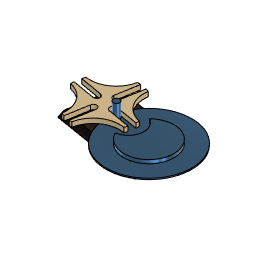
cool_old_stuffff (Autodesk Fusion 360 design; units mm, degrees)
Autodesk Fusion 360 part; units mm, degrees
sketch "Sketch1" plane through (0, 0, 0) normal (0, 0, 1) x (1, 0, 0)
  line L0 (70, 40) -> (-70, 40)
  line L1 (-70, 40) -> (-70, -40)
  line L2 (-70, -40) -> (70, -40)
  line L3 (70, -40) -> (70, 40)
  line L4 (70, 40) -> (-70, -40) construction
  line L5 (-70, 40) -> (70, -40) construction
  constraint horizontal L0
  constraint perpendicular L0 L1
  constraint parallel L0 L2
  constraint parallel L1 L3
  constraint coincident L4 origin
  constraint coincident L5 origin
ref_plane "WorkPlane1" through (0, 0, 10) normal (0, 0, 1) x (1, 0, 0)
sketch "Sketch2" plane through (0, 0, 10) normal (0, 0, 1) x (1, 0, 0)
  line L0 (65, -35) -> (-65, -35)
  line L1 (-65, -35) -> (-65, 35)
  line L2 (-65, 35) -> (65, 35)
  line L3 (65, 35) -> (65, -35)
  line L4 (65, -35) -> (-65, 35) construction
  line L5 (-65, -35) -> (65, 35) construction
  constraint horizontal L0
  constraint perpendicular L0 L1
  constraint parallel L0 L2
  constraint parallel L1 L3
  constraint coincident L4 origin
  constraint coincident L5 origin
loft "Loft1" add profiles "Sketch1", "Sketch2" section 1 section 2 makes body 1
sketch "Sketch3" plane through (0, 0, 10) normal (0, 0, 1) x (-1, 0, 0)
  line L0 (-65, 35) -> (-65, -35)
  line L1 (-65, -35) -> (65, -35)
  line L2 (65, -35) -> (65, 35)
  line L3 (65, 35) -> (-65, 35)
  circle A0 centre (40, 0) radius 7.5
  circle A1 centre (-40, 0) radius 7.5
  dimension "d2" = 15
  dimension "d3" = 15
  measures "d2" diameter of A0
  measures "d3" diameter of A1
extrude "Extrude1" cut sketch "Sketch3" against normal blind 35 contours A0 | A1 bodies 1
sketch "Sketch5" plane through (0, 0, 10) normal (0, 0, 1) x (1, 0, 0)
  line L0 (-54.9257, 4.9994) -> (-89.7494, 4.9994)
  line L1 (-54.9257, -4.9994) -> (-89.7494, -4.9994)
  line L2 (-44.9992, 14.9113) -> (-44.9992, 49.7495)
  line L3 (-35.0008, 14.9113) -> (-35.0008, 49.7495)
  line L4 (-25.0347, 4.9999) -> (9.7494, 4.9999)
  line L5 (-25.0347, -4.9999) -> (9.7494, -4.9999)
  line L6 (-35.0004, -14.9355) -> (-35.0004, -49.7494)
  line L7 (-44.9996, -14.9355) -> (-44.9996, -49.7494)
  arc A0 (-55.0743, -4.9994) -> (-55.0743, 4.9994) centre (-55, 0) ccw
  arc A1 (-44.9992, 15.0887) -> (-35.0008, 15.0887) centre (-40, 15) ccw
  arc A2 (-24.9653, 4.9999) -> (-24.9653, -4.9999) centre (-25, 0) ccw
  arc A3 (-35.0004, -15.0645) -> (-44.9996, -15.0645) centre (-40, -15) ccw
  line L8 (-44.9996, -49.7494) -> (-104, -49) construction
  line L9 (-104, -49) -> (-93.0357, -49.1393) construction
  line L10 (-89.7494, -4.9994) -> (-89.7494, -49.181) construction
  line L11 (-89.7494, 4.9994) -> (-89.7494, 62) construction
  line L12 (-89.7494, 62) -> (-72.3376, 62) construction
  line L13 (-72.3376, 62) -> (-89.7494, 58.8778) construction
  line L14 (-53.6946, 49.7495) -> (-91, 49.7495) construction
  line L15 (-91, 49.7495) -> (-87, 49.7495) construction
  line L16 (-35.0008, 49.7495) -> (24, 49.7495) construction
  line L17 (24, 49.7495) -> (20, 49.7495) construction
  line L18 (9.7494, 4.9999) -> (10, 52) construction
  line L19 (10, 52) -> (9.988, 49.7495) construction
  line L20 (9.7494, -4.9999) -> (9.7494, -65) construction
  line L21 (9.7494, -65) -> (9.7494, -62) construction
  line L22 (-35.0004, -49.7494) -> (11, -49.7494) construction
  line L23 (11, -49.7494) -> (9.7494, -49.7494) construction
  arc A4 (-49.7527, -49.689) -> (-89.7494, -9.181) centre (-89.7494, -49.181) ccw
  arc A5 (-89.7494, -4.9994) -> (-89.149, -9.1855) centre (-40, 0) ccw
  arc A6 (-49.7497, -49.0402) -> (-44.9996, -49.7494) centre (-40, 0) ccw
  arc A7 (-89.7494, 9.7495) -> (-49.7557, 49.039) centre (-89.7494, 49.7495) ccw
  arc A8 (-44.9992, 49.7495) -> (-49.7557, 49.039) centre (-40, 0) ccw
  arc A9 (-89.039, 9.7558) -> (-89.7494, 4.9994) centre (-40, 0) ccw
  arc A10 (-30.012, 49.7495) -> (9.7747, 9.75) centre (9.988, 49.7495) ccw
  arc A11 (9.7494, 4.9999) -> (9.038, 9.7607) centre (-40, 0) ccw
  arc A12 (-30.0048, 48.9908) -> (-35.0008, 49.7495) centre (-40, 0) ccw
  arc A13 (9.7494, -9.7494) -> (-30.2506, -49.7494) centre (9.7494, -49.7494) ccw
  arc A14 (-35.0004, -49.7494) -> (-30.2443, -49.039) centre (-40, 0) ccw
  arc A15 (9.039, -9.7557) -> (9.7494, -4.9999) centre (-40, 0) ccw
  dimension "d15" = 100
  dimension "d16" = 10
  dimension "d17" = 10
  dimension "d18" = 10
  dimension "d19" = 10
  dimension "d20" = 80
  dimension "d21" = 80
  dimension "d22" = 80
  dimension "d23" = 80
  constraint coincident L0.start A0
  constraint horizontal L0
  constraint coincident L1.start A0
  constraint parallel L0 L1
  constraint coincident L2.start A1
  constraint coincident L2.end A5
  constraint perpendicular L1 L2
  constraint coincident L3.start A1
  constraint parallel L2 L3
  constraint coincident L4.start A2
  constraint coincident L4.end A5
  constraint perpendicular L3 L4
  constraint coincident L5.start A2
  constraint perpendicular L3 L5
  constraint coincident L6.start A3
  constraint coincident L6.end A5
  constraint perpendicular L0 L6
  constraint coincident L7.start A3
  constraint parallel L6 L7
  constraint coincident L0 A0.end
  constraint coincident L1 A0.start
  constraint coincident L3 A1.end
  constraint coincident L2 A1.start
  constraint concentric A5 A8
  constraint coincident L5 A2.end
  constraint coincident L4 A2.start
  constraint concentric A5 A11
  constraint coincident L7 A3.end
  constraint coincident L6 A3.start
  constraint concentric A5 A14
  constraint coincident L8 L9.end
  constraint parallel L8 L9
  constraint coincident L8 L10.end
  constraint perpendicular L1 L10
  constraint perpendicular L0 L11
  constraint perpendicular L11 L12
  constraint coincident L11 L13.end
  constraint perpendicular L11 L14
  constraint coincident L14 L15.end
  constraint perpendicular L11 L15
  constraint perpendicular L3 L16
  constraint coincident L16 L17.end
  constraint perpendicular L3 L17
  constraint coincident L18 L19.end
  constraint coincident L16 L19.end
  constraint parallel L18 L19
  constraint perpendicular L5 L20
  constraint coincident L20 L21.end
  constraint perpendicular L5 L21
  constraint perpendicular L20 L22
  constraint coincident L22 L23.end
  constraint coincident L20 L23.end
  constraint perpendicular L20 L23
  constraint coincident L10.end A4.centre
  constraint coincident L14 A7.centre
  constraint coincident L11 A7.centre
  constraint coincident L19.end A10.centre
  constraint coincident L10 A4.end
  constraint coincident L8 A4.start
  constraint coincident A4 A5.end
  constraint coincident A4 A6.start
  constraint concentric A5 A6
  constraint coincident L11 A7.start
  constraint coincident A7 A9.start
  constraint concentric A8 A9
  constraint coincident L18 A10.end
  constraint coincident L16 A10.start
  constraint coincident A10 A11.end
  constraint coincident A10 A12.start
  constraint concentric A11 A12
  constraint coincident L23.end A13.centre
  constraint coincident L22 A13.end
  constraint coincident L20 A13.start
  constraint coincident A13 A14.end
  constraint coincident A13 A15.start
  constraint concentric A14 A15
  measures "d15" diameter of A5
  measures "d16" diameter of A0
  measures "d17" diameter of A1
  measures "d18" diameter of A2
  measures "d19" diameter of A3
  measures "d20" diameter of A4
  measures "d21" diameter of A7
  measures "d22" diameter of A10
  measures "d23" diameter of A13
ref_plane "WorkPlane3" through (0, 0, 20) normal (0, 0, 1) x (-1, 0, 0)
sketch "Sketch7" plane through (0, 0, 20) normal (0, 0, 1) x (1, 0, 0)
  line L0 (-54.7838, 4.9953) -> (-89.7498, 4.9953)
  line L1 (-54.7838, -4.9953) -> (-89.7498, -4.9953)
  line L2 (-44.998, 15.1402) -> (-44.998, 49.7496)
  line L3 (-35.002, 15.1402) -> (-35.002, 49.7496)
  line L4 (-24.9087, 4.9992) -> (9.7495, 4.9992)
  line L5 (-24.9087, -4.9992) -> (9.7495, -4.9992)
  line L6 (-45, -14.9847) -> (-45.1061, -49.7386)
  line L7 (-35, -14.9847) -> (-34.8939, -49.7386)
  arc A0 (-88.9872, 10.0128) -> (-50.0128, 48.9872) centre (-90, 50) ccw
  arc A1 (-44.998, 49.7496) -> (-50.0128, 48.9872) centre (-40, 0) ccw
  arc A2 (-44.998, 15.1402) -> (-35.002, 15.1402) centre (-40, 15) ccw
  arc A3 (-29.9872, 48.9872) -> (8.9872, 10.0128) centre (10, 50) ccw
  arc A4 (-29.9872, 48.9872) -> (-35.002, 49.7496) centre (-40, 0) ccw
  arc A5 (9.7495, 4.9992) -> (8.9872, 10.0128) centre (-40, 0) ccw
  arc A6 (-24.9087, 4.9992) -> (-24.9087, -4.9992) centre (-25, 0) ccw
  arc A7 (8.9872, -10.0128) -> (-29.9872, -48.9872) centre (10, -50) ccw
  arc A8 (8.9872, -10.0128) -> (9.7495, -4.9992) centre (-40, 0) ccw
  arc A9 (-34.8939, -49.7386) -> (-29.9872, -48.9872) centre (-40, 0) ccw
  arc A10 (-35, -14.9847) -> (-45, -14.9847) centre (-40, -15) ccw
  arc A11 (-50, -48.9898) -> (-89.1818, -9.0084) centre (-90, -49) ccw
  arc A12 (-50, -48.9898) -> (-45.1061, -49.7386) centre (-40, 0) ccw
  arc A13 (-88.9872, 10.0128) -> (-89.7498, 4.9953) centre (-40, 0) ccw
  arc A14 (-89.7498, -4.9953) -> (-89.1818, -9.0084) centre (-40, 0) ccw
  arc A15 (-55.2162, -4.9953) -> (-55.2162, 4.9953) centre (-55, 0) ccw
  dimension "d25" = 100
  dimension "d26" = 80
  dimension "d27" = 80
  dimension "d28" = 80
  dimension "d29" = 80
  dimension "d30" = 10
  dimension "d31" = 10
  dimension "d32" = 10
  dimension "d33" = 10
  constraint coincident L0.start A15
  constraint horizontal L0
  constraint coincident L1.start A15
  constraint coincident L1.end A13
  constraint parallel L0 L1
  constraint coincident L2.end A13
  constraint perpendicular L0 L2
  constraint parallel L2 L3
  constraint coincident L4.end A13
  constraint perpendicular L3 L4
  constraint parallel L4 L5
  constraint tangent L6 A10
  constraint coincident L7.end A13
  constraint tangent L7 A10
  constraint concentric A1 A13
  constraint coincident A3.start A13
  constraint concentric A4 A13
  constraint concentric A5 A13
  constraint coincident A7.start A13
  constraint concentric A8 A13
  constraint concentric A9 A13
  constraint coincident A11.start A13
  constraint concentric A12 A13
  constraint concentric A13 A14
  constraint coincident L0 A15.end
  constraint coincident L1 A15.start
  measures "d25" diameter of A13
  measures "d26" diameter of A0
  measures "d27" diameter of A3
  measures "d28" diameter of A7
  measures "d29" diameter of A11
  measures "d30" diameter of A15
  measures "d31" diameter of A2
  measures "d32" diameter of A6
  measures "d33" diameter of A10
extrude "Extrude1'" add sketch "Sketch7" against normal blind 7 separate body contours L0 L1 L2 L3 L4 L5 L6 L7 A0 A1 A2 A3 A4 A5 A6 A7 A8 A9 A10 A11 A12 A13 A14 A15 makes body 2 in component "rotita"
sketch "Sketch8" plane through (0, 0, 20) normal (0, 0, 1) x (-1, 0, 0)
  arc A0 (89.7498, 4.9953) -> (89.1818, 9.0084) centre (40, 0) ccw
  arc A1 (50, 48.9898) -> (89.1818, 9.0084) centre (90, 49) ccw
  arc A2 (50, 48.9898) -> (45.1061, 49.7386) centre (40, 0) ccw
  line L0 (45.1061, 49.7386) -> (45, 14.9847)
  arc A3 (35, 14.9847) -> (45, 14.9847) centre (40, 15) ccw
  line L1 (35, 14.9847) -> (34.8939, 49.7386)
  arc A4 (34.8939, 49.7386) -> (29.9872, 48.9872) centre (40, 0) ccw
  arc A5 (-8.9872, 10.0128) -> (29.9872, 48.9872) centre (-10, 50) ccw
  arc A6 (-8.9872, 10.0128) -> (-9.7495, 4.9992) centre (40, 0) ccw
  line L2 (-9.7495, 4.9992) -> (24.9087, 4.9992)
  arc A7 (24.9087, -4.9992) -> (24.9087, 4.9992) centre (25, 0) ccw
  line L3 (24.9087, -4.9992) -> (-9.7495, -4.9992)
  arc A8 (-9.7495, -4.9992) -> (-8.9872, -10.0128) centre (40, 0) ccw
  arc A9 (29.9872, -48.9872) -> (-8.9872, -10.0128) centre (-10, -50) ccw
  arc A10 (29.9872, -48.9872) -> (35.002, -49.7496) centre (40, 0) ccw
  line L4 (35.002, -49.7496) -> (35.002, -15.1402)
  arc A11 (44.998, -15.1402) -> (35.002, -15.1402) centre (40, -15) ccw
  line L5 (44.998, -15.1402) -> (44.998, -49.7496)
  arc A12 (44.998, -49.7496) -> (50.0128, -48.9872) centre (40, 0) ccw
  arc A13 (88.9872, -10.0128) -> (50.0128, -48.9872) centre (90, -50) ccw
  arc A14 (88.9872, -10.0128) -> (89.7498, -4.9953) centre (40, 0) ccw
  line L6 (89.7498, -4.9953) -> (55.2162, -4.9953)
  arc A15 (55.2162, 4.9953) -> (55.2162, -4.9953) centre (55, 0) ccw
  line L7 (55.2162, 4.9953) -> (89.7498, 4.9953)
  circle A16 centre (40, 0) radius 6
  dimension "d36" = 12
  constraint concentric A0 A16
  measures "d36" diameter of A16
extrude "Extrude2" add sketch "Sketch8" against normal blind 20 contours A16 bodies 2 in component "rotita"
ref_plane "WorkPlane4" through (0, 0, 13) normal (0, 0, 1) x (-1, 0, 0)
sketch "Sketch9" plane through (0, 0, 13) normal (0, 0, 1) x (1, 0, 0)
ref_plane "WorkPlane5" through (0, 0, 11) normal (0, 0, 1) x (-1, 0, 0)
sketch "Sketch10" plane through (0, 0, 11) normal (0, 0, 1) x (1, 0, 0)
  circle A0 centre (40, 0) radius 64.0819
  arc A1 (9.8689, -22.3241) -> (9.8573, 22.3085) centre (2.5, -0.0097) ccw
  arc A2 (9.8689, -22.3241) -> (9.8573, 22.3085) centre (40, 0) ccw
  circle A3 centre (-19, 0) radius 4.85
  dimension "d41" = 75
  dimension "d42" = 9.7
  constraint concentric A0 A2
  constraint coincident A1.centre A2
  measures "d41" diameter of A2
  measures "d42" diameter of A3
extrude "Extrude2'" add sketch "Sketch10" along normal blind 1.8 separate body contours A0 | A1 A2 | A3 makes body 3
extrude "Extrude3" add sketch "Sketch10" along normal blind 7.2 contours A1 A2 bodies 3
extrude "Extrude4" add sketch "Sketch10" along normal blind 23 contours A3 bodies 3
copy_body "Body->Comp1" bodies 3 removing the originals makes body 4 in component "Component"
copy_body "Body->Comp2" bodies 1 removing the originals makes body 5 in component "suport"
sketch "Sketch11" plane through (0, 0, 12.8) normal (0, 0, 1) x (-1, 0, 0)
  circle A0 centre (19, 0) radius 4.85
  arc A1 (-9.8689, 22.3241) -> (-9.8573, -22.3085) centre (-2.5, 0.0097) ccw
  arc A2 (-9.8689, 22.3241) -> (-9.8573, -22.3085) centre (-40, 0) ccw
  circle A3 centre (-40, 0) radius 64.0819
  circle A4 centre (-40, 0) radius 6
  dimension "d49" = 12
  constraint concentric A2 A4
  measures "d49" diameter of A4
extrude "Extrude1''" add sketch "Sketch11" against normal blind 12.8 contours A4 bodies 4 in component "Component"
component "rotita" placed x (-1, 0, 0) y (0, -1, 0) z (0, 0, 1) at (-80.0002, 0.0055, 0)
component "Component" placed x (1, 0, 0) y (0, 1, 0) z (0, 0, 1) at (0, 0, 0)
component "suport" placed x (1, 0, 0) y (0, 1, 0) z (0, 0, 1) at (0, 0, 0)
named bodies: "suport"
